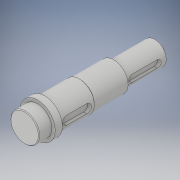
# Autodesk Inventor part: hridel
Saved by Autodesk Inventor 2019 (Build 230136000, 136)
## iProperties
Created: 2020-06-01
Part Number: hridel
Material: Všeobecné
Document SubType Name: Modeling
Designer: hynek
Density: 1 g/cm^3
Appearance: Výchozí
Author: hynek
Autodesk Inventor part; units mm, degrees
ref_plane "YZ Plane" through (0, 0, 0) normal (1, 0, 0) x (0, 1, 0)
ref_plane "XZ Plane" through (0, 0, 0) normal (0, 1, 0) x (-1, 0, 0)
ref_plane "XY Plane" through (0, 0, 0) normal (0, 0, 1) x (1, 0, 0)
sketch "Náčrt1" plane through (0, 0, 0) normal (0, 0, 1) x (1, 0, 0)
  circle A0 centre (0, 0) radius 24.5
  dimension "d0" = 49
  constraints: 1 centre point, 1 coincident
  measures "d0" diameter of A0
extrude "Vysunutí1" add sketch "Náčrt1" along normal mid plane 10
sketch "Náčrt2" plane through (0, 0, 5) normal (0, 0, 1) x (1, 0, 0)
  circle A0 centre (0, 0) radius 20
  dimension "d3" = 40
  constraints: 1 centre point, 1 coincident
  measures "d3" diameter of A0
extrude "Vysunutí2" add sketch "Náčrt2" along normal blind 18
sketch "Náčrt3" plane through (0, 0, -5) normal (0, 0, -1) x (-1, 0, 0)
  circle A0 centre (0, 0) radius 21
  dimension "d6" = 42
  constraints: 1 centre point, 1 coincident
  measures "d6" diameter of A0
extrude "Vysunutí3" add sketch "Náčrt3" along normal blind 48
sketch "Náčrt4" plane through (0, 0, -53) normal (0, 0, -1) x (-1, 0, 0)
  circle A0 centre (0, 0) radius 20
  dimension "d9" = 40
  constraints: 1 centre point, 1 coincident
  measures "d9" diameter of A0
extrude "Vysunutí4" add sketch "Náčrt4" along normal blind 48
sketch "Náčrt5" plane through (0, 0, -101) normal (0, 0, -1) x (-1, 0, 0)
  circle A0 centre (0, 0) radius 16
  dimension "d12" = 32
  constraints: 1 centre point, 1 coincident
  measures "d12" diameter of A0
extrude "Vysunutí5" add sketch "Náčrt5" along normal blind 58
sketch "Náčrt6" plane through (0, 0, 0) normal (1, 0, 0) x (0, 1, 0)
  line L0 (0, -9) -> (0, -49) construction
  line L1 (-6, -15) -> (-6, -43)
  line L2 (6, -43) -> (6, -15)
  arc A0 (6, -15) -> (-6, -15) centre (0, -15) ccw
  arc A1 (-6, -43) -> (6, -43) centre (0, -43) ccw
  line L3 (-24.5, -5) -> (24.5, -5) projected
  line L4 (0, -195.4) -> (0, 59.4) projected
  line L5 (-21, -53) -> (21, -53) projected
  point P0 (0, 0)
  point P1 (0, -29)
  dimension "d15" = 12
  dimension "d16" = 4
  dimension "d17" = 4
  constraints: 8 end point, 6 point on circle, 4 tangent, 3 point on line, 2 centre point, 1 midpoint, 1 parallel, 1 vertical
  measures "d15" distance between parallel lines of L2 L1
  measures "d16" distance from line of L3 L0.start
  measures "d17" distance from line of L5 L0.end
extrude "Vysunutí6" cut sketch "Náčrt6" along normal through all
sketch "Náčrt7" plane through (0, 0, 0) normal (1, 0, 0) x (0, 0, -1)
  line L0 (15, -6) -> (43, -6) projected
  arc A0 (43, -6) -> (43, 6) centre (43, 0) ccw projected
  line L1 (43, 6) -> (15, 6) projected
  arc A1 (15, 6) -> (15, -6) centre (15, 0) ccw projected
  point P0 (0, 0)
extrude "Vysunutí7" add sketch "Náčrt7" along normal blind 16.1 and the other way blind 18.55
sketch "Náčrt8" plane through (0, 0, 0) normal (1, 0, 0) x (0, 1, 0)
  line L0 (0, -195.4) -> (0, 59.4) projected
  line L1 (0, -106) -> (0, -151) construction
  line L2 (-5, -111) -> (-5, -146)
  line L3 (5, -146) -> (5, -111)
  arc A0 (5, -111) -> (-5, -111) centre (0, -111) ccw
  arc A1 (-5, -146) -> (5, -146) centre (0, -146) ccw
  line L4 (-20, -101) -> (20, -101) projected
  point P0 (0, 0)
  point P1 (0, -128.5)
  dimension "d24" = 10
  dimension "d25" = 5
  dimension "d26" = 35
  constraints: 8 end point, 6 point on circle, 4 point on line, 4 tangent, 2 centre point, 1 midpoint, 1 parallel
  measures "d24" distance between parallel lines of L3 L2
  measures "d25" distance from line of L4 L1.start
  measures "d26" distance of L2.start L2.end
extrude "Vysunutí8" cut sketch "Náčrt8" along normal through all
sketch "Náčrt9" plane through (0, 0, 0) normal (1, 0, 0) x (0, 0, -1)
  line L0 (111, -5) -> (146, -5) projected
  arc A0 (146, -5) -> (146, 5) centre (146, 0) ccw projected
  line L1 (146, 5) -> (111, 5) projected
  arc A1 (111, 5) -> (111, -5) centre (111, 0) ccw projected
  point P0 (0, 0)
extrude "Vysunutí9" add sketch "Náčrt9" along normal blind 11.3
chamfer "Zkosení1" distance 1 angle 45 1 edges at (-20, 0, 23)
fillet "Zaoblení2" radius 1 3 edges at (21, 0, -5) (20, 0, -53) (16, 0, -159)
fillet "Zaoblení2" radius 2.5 1 edges at (16, 0, -101)
